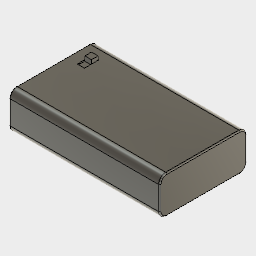
727 3x AAA Battery Holder (Autodesk Fusion 360 design; units mm, degrees)
Autodesk Fusion 360 part; units mm, degrees
sketch "Sketch1" plane through (0, 0, 0) normal (0, 0, 1) x (1, 0, 0)
  line L0 (0, 0) -> (64, 0)
  line L1 (64, 0) -> (64, 37)
  line L2 (64, 37) -> (0, 37)
  line L3 (0, 37) -> (0, 0)
  dimension "d1" = 64
  dimension "d2" = 37
  measures "d1" distance of L1.end L2.end
  measures "d2" distance of L0.end L1.end
extrude "Extrude1" add sketch "Sketch1" along normal blind 16
fillet "Fillet1" radius 3 4 edges at (32, 0, 16) (32, 37, 16) (32, 0, 0) (32, 37, 0)
fillet "Fillet2" radius 0.5 16 edges at (64, 36.1213, 0.8787) (64, 37, 8) (64, 36.1213, 15.1213) (64, 18.5, 16) (64, 0.8787, 15.1213) (64, 0, 8) (64, 0.8787, 0.8787) (64, 18.5, 0) (0, 0.8787, 0.8787) (0, 0, 8) (0, 0.8787, 15.1213) (0, 18.5, 16) (0, 36.1213, 15.1213) (0, 37, 8) (0, 36.1213, 0.8787) (0, 18.5, 0)
sketch "Sketch2" plane through (0, 0, 16) normal (0, 0, 1) x (-1, 0, 0)
  line L0 (-0.5, -34) -> (-0.5, -3)
  line L1 (-0.5, -3) -> (-63.5, -3)
  line L2 (-63.5, -3) -> (-63.5, -34)
  line L3 (-63.5, -34) -> (-0.5, -34)
  line L4 (-5, -24) -> (-8, -24)
  line L5 (-8, -24) -> (-8, -30)
  line L6 (-8, -30) -> (-5, -30)
  line L7 (-5, -30) -> (-5, -24)
  dimension "d7" = 3
  dimension "d8" = 6
  measures "d7" distance of L4.start L4.end
  measures "d8" distance of L4.start L6.end
extrude "Extrude2" cut sketch "Sketch2" against normal blind 0.5 contours L4 L5 L6 L7
sketch "Sketch3" plane through (0, 0, 15.5) normal (0, 0, 1) x (-1, 0, 0)
  line L0 (-5, -30) -> (-5, -24)
  line L1 (-5, -24) -> (-8, -24)
  line L2 (-8, -24) -> (-8, -30)
  line L3 (-8, -30) -> (-5, -30)
  line L4 (-5, -27) -> (-8, -27)
  line L5 (-5.1, -27.1) -> (-7.9, -27.1)
  line L6 (-7.9, -27.1) -> (-7.9, -29.9)
  line L7 (-7.9, -29.9) -> (-5.1, -29.9)
  line L8 (-5.1, -29.9) -> (-5.1, -27.1)
extrude "Extrude3" add sketch "Sketch3" along normal blind 2 contours L5 L6 L7 L8
